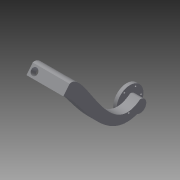
# Autodesk Inventor part: fork
Saved by Autodesk Inventor 2013 (Build 170138000, 138)
## iProperties
Created: 2013-01-09
Part Number: fork
Material: Generic
Document SubType Name: Modeling
Designer: Nano
Density: 1 g/cm^3
Author: Nano
Autodesk Inventor part; units mm, degrees
ref_plane "YZ Plane" through (0, 0, 0) normal (1, 0, 0) x (0, 1, 0)
ref_plane "XZ Plane" through (0, 0, 0) normal (0, 1, 0) x (-1, 0, 0)
ref_plane "XY Plane" through (0, 0, 0) normal (0, 0, 1) x (1, 0, 0)
sketch "Sketch1" plane through (0, 0, 0) normal (1, 0, 0) x (0, 1, 0)
  circle A0 centre (-479.4213, -671.0964) radius 25.4
  circle A1 centre (-479.4213, -671.0964) radius 88.9 projected
  circle A2 centre (-479.4213, -649.9452) radius 1.5875
  circle A3 centre (-497.7388, -660.5208) radius 1.5875
  circle A4 centre (-497.7388, -681.6721) radius 1.5875
  circle A5 centre (-479.4213, -692.2477) radius 1.5875
  circle A6 centre (-461.1038, -681.6721) radius 1.5875
  circle A7 centre (-461.1038, -660.5208) radius 1.5875
  point P0 (0, 0)
  dimension "d0" = 50.8
  dimension "d1" = 3.175
  dimension "d4" = 360
  constraints: 7 centre point, 1 concentric, 13 other
  measures "d0" diameter of A0
  measures "d1" diameter of A2
extrude "Extrusion1" add sketch "Sketch1" along normal blind 6.35 contours A0
sketch "Sketch2" plane through (6.35, -479.4213, -671.0964) normal (1, 0, 0) x (0, 0, -1)
  circle A0 centre (-21.1512, 0) radius 1.5875 projected
  spline S0 degree 3 poles (-5.6187, -9.891) (-73.0206, -34.6538) (-119.0516, 78.5765) (-145.3355, 88.8855) knots 0 0 0 0 1 1 1 1
  spline S1 degree 3 poles (0, 11.5539) (-60.9983, -36.2975) (-102.9311, 114.869) (-133.6383, 103.832) knots 0 0 0 0 1 1 1 1
  line L0 (-145.3355, 88.8855) -> (-133.6383, 103.832)
  arc A1 (-5.6187, -9.891) -> (0, 11.5539) centre (0.2097, 0.0404) ccw
  point P0 (-671.0964, 479.4213)
  point P1 (-69.3034, 5.0557)
  point P2 (-121.2912, 64.8414)
  point P3 (-55.007, 16.7301)
  point P4 (-109.594, 88.8855)
  constraints: 2 end point, 2 point on circle, 1 centre point, 8 other
extrude "Extrusion2" add sketch "Sketch2" along normal blind 19.05
sketch "Sketch3" plane through (6.35, -479.4213, -671.0964) normal (-1, 0, 0) x (0, 0, 1)
  spline S0 degree 3 poles (21.6253, -13.3232) (80.3701, -16.9336) (121.1871, 79.4141) (145.3355, 88.8855) knots 0 0 0 0 1 1 1 1 projected
  line L0 (145.3355, 88.8855) -> (133.6383, 103.832) projected
  spline S1 degree 3 poles (133.6383, 103.832) (107.3744, 113.2719) (72.8986, 4.0539) (25.3056, 2.1884) knots 0 0 0 0 1 1 1 1 projected
  line L1 (135.1558, 81.2846) -> (120.3749, 100.1713)
  point P0 (671.0964, 479.4213)
  constraints: 2 end point, 1 parallel, 4 other
extrude "Extrusion3" add sketch "Sketch3" along normal blind 50.8
sketch "Sketch4" plane through (-44.45, -375.5893, -537.4582) normal (0, 0.6163082, 0.787505) x (1, 0, 0)
  line L0 (50.8, -18.9795) -> (0, -18.9795) projected
  spline S0 degree 4 poles (22.0839, 128.199) (22.0839, 128.1731) (22.0839, 75.9092) (22.0839, -57.7492) (22.0839, -145.2754) (22.0839, -219.2952) (22.0839, -161.3853) (22.0839, -142.8391) knots 0 0 0 0 0 0.294993 0.49649 0.669634 1 1 1 1 1 projected
  spline S1 degree 4 poles (-3.3161, -142.8391) (-3.3161, -161.3853) (-3.3161, -219.2952) (-3.3161, -145.2754) (-3.3161, -57.7492) (-3.3161, 75.9092) (-3.3161, 128.1731) (-3.3161, 128.199) knots -1 -1 -1 -1 -1 -0.669634 -0.49649 -0.294993 0 0 0 0 0 projected
  line L1 (-3.3161, 128.199) -> (22.0839, 128.199) construction
  line L2 (9.3839, 128.199) -> (9.3839, -142.8391) construction
  circle A0 centre (9.3839, -9.4897) radius 6.35
  point P0 (44.45, -35.4614)
  dimension "d12" = 12.7
  constraints: 4 end point, 1 centre point, 1 midpoint, 1 parallel, 1 perpendicular, 1 point on line
  measures "d12" diameter of A0
extrude "Extrusion4" cut sketch "Sketch4" against normal through all
body "Solid1"
